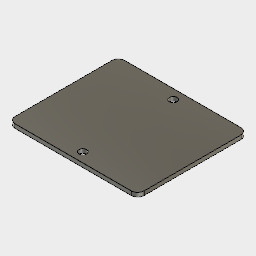
1608 perma-proto quarter (Autodesk Fusion 360 design; units mm, degrees)
Autodesk Fusion 360 part; units mm, degrees
sketch "Sketch1" plane through (0, 0, 0) normal (0, 0, 1) x (1, 0, 0)
  line L0 (0, 0) -> (50.8, 0)
  line L1 (50.8, 0) -> (50.8, 43.18)
  line L2 (50.8, 43.18) -> (0, 43.18)
  line L3 (0, 43.18) -> (0, 0)
  line L4 (25.4, 43.18) -> (25.4, 0) construction
  line L5 (0, 21.59) -> (50.8, 21.59) construction
  circle A0 centre (25.4, 39.37) radius 1.5
  circle A1 centre (25.4, 3.81) radius 1.5
  dimension "d1" = 50.8
  dimension "d2" = 43.18
  dimension "d3" = 3
  dimension "d4" = 3
  dimension "d5" = 17.78
  dimension "d6" = 35.56
  measures "d1" distance of L0.start L0.end
  measures "d2" distance of L0.start L2.end
  measures "d3" diameter of A0
  measures "d4" diameter of A1
  measures "d5" distance of L5 A0.centre
  measures "d6" distance of A0.centre A1.centre
extrude "Extrude1" add sketch "Sketch1" along normal blind 1.6
fillet "Fillet1" radius 2.54 4 edges at (50.8, 0, 0.8) (50.8, 43.18, 0.8) (0, 0, 0.8) (0, 43.18, 0.8)
